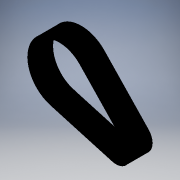
# Autodesk Inventor part: ベルト
Saved by Autodesk Inventor 2022 (Build 260153000, 153)
## iProperties
Created: 2021-07-07
Part Number: ベルト
Material: 一般
Document SubType Name: Modeling
Designer: nrz71
Density: 1 g/cm^3
Appearance: 既定
Author: nrz71
Autodesk Inventor part; units mm, degrees
ref_plane "YZ Plane" through (0, 0, 0) normal (1, 0, 0) x (0, 1, 0)
ref_plane "XZ Plane" through (0, 0, 0) normal (0, 1, 0) x (-1, 0, 0)
ref_plane "XY Plane" through (0, 0, 0) normal (0, 0, 1) x (1, 0, 0)
sketch "スケッチ1" plane through (0, 0, 0) normal (0, 0, 1) x (1, 0, 0)
  circle A0 centre (0, 0) radius 4.5
  circle A1 centre (0, 0) radius 3.5
  circle A2 centre (-17.9655, 10.8739) radius 0.9295 projected
  arc A3 (-15.3759, 19.6478) -> (-15.5156, 19.8402) centre (-15.5657, 19.657) ccw projected
  arc A4 (-15.5156, 19.8402) -> (-15.828, 19.9198) centre (-17.9655, 10.8739) ccw projected
  arc A5 (-15.828, 19.9198) -> (-16.0427, 19.8177) centre (-15.8717, 19.7349) ccw projected
  arc A6 (-16.4782, 19.3076) -> (-16.0427, 19.8177) centre (-17.2354, 20.3949) ccw projected
  arc A7 (-16.5519, 19.291) -> (-16.4782, 19.3076) centre (-16.5354, 19.3896) ccw projected
  arc A8 (-16.5519, 19.291) -> (-16.9189, 19.3445) centre (-17.9655, 10.8739) ccw projected
  arc A9 (-16.9848, 19.3814) -> (-16.9189, 19.3445) centre (-16.9067, 19.4437) ccw projected
  arc A10 (-17.2567, 19.9945) -> (-16.9848, 19.3814) centre (-15.9489, 20.2075) ccw projected
  arc A11 (-17.2567, 19.9945) -> (-17.4334, 20.1537) centre (-17.4442, 19.964) ccw projected
  arc A12 (-17.4334, 20.1537) -> (-17.7555, 20.1665) centre (-17.9655, 10.8739) ccw projected
  arc A13 (-17.7555, 20.1665) -> (-17.9443, 20.022) centre (-17.7598, 19.9766) ccw projected
  arc A14 (-18.2642, 19.4325) -> (-17.9443, 20.022) centre (-19.2309, 20.3387) ccw projected
  arc A15 (-18.3328, 19.401) -> (-18.2642, 19.4325) centre (-18.3371, 19.5009) ccw projected
  arc A16 (-18.3328, 19.401) -> (-18.7029, 19.377) centre (-17.9655, 10.8739) ccw projected
  arc A17 (-18.7751, 19.3994) -> (-18.7029, 19.377) centre (-18.7116, 19.4766) ccw projected
  arc A18 (-19.1685, 19.9426) -> (-18.7751, 19.3994) centre (-17.9336, 20.4228) ccw projected
  arc A19 (-19.1685, 19.9426) -> (-19.3744, 20.0615) centre (-19.3456, 19.8737) ccw projected
  arc A20 (-19.3744, 20.0615) -> (-19.6921, 20.0071) centre (-17.9655, 10.8739) ccw projected
  arc A21 (-19.6921, 20.0071) -> (-19.8467, 19.8265) centre (-19.6568, 19.8204) ccw projected
  arc A22 (-20.0371, 19.1834) -> (-19.8467, 19.8265) centre (-21.171, 19.8688) ccw projected
  arc A23 (-20.0977, 19.1383) -> (-20.0371, 19.1834) centre (-20.1227, 19.2351) ccw projected
  arc A24 (-20.0977, 19.1383) -> (-20.4547, 19.0378) centre (-17.9655, 10.8739) ccw projected
  arc A25 (-20.5299, 19.0447) -> (-20.4547, 19.0378) centre (-20.4839, 19.1335) ccw projected
  arc A26 (-21.0277, 19.4943) -> (-20.5299, 19.0447) centre (-19.9196, 20.2208) ccw projected
  arc A27 (-21.0277, 19.4943) -> (-21.2538, 19.5678) centre (-21.1866, 19.3901) ccw projected
  arc A28 (-21.2538, 19.5678) -> (-21.5533, 19.4485) centre (-17.9655, 10.8739) ccw projected
  arc A29 (-21.5533, 19.4485) -> (-21.667, 19.2397) centre (-21.4799, 19.2733) ccw projected
  arc A30 (-21.7195, 18.5711) -> (-21.667, 19.2397) centre (-22.9711, 19.0057) ccw projected
  arc A31 (-21.7694, 18.5144) -> (-21.7195, 18.5711) centre (-21.8139, 18.6039) ccw projected
  arc A32 (-21.7694, 18.5144) -> (-22.0977, 18.3419) centre (-17.9655, 10.8739) ccw projected
  arc A33 (-22.1727, 18.333) -> (-22.0977, 18.3419) centre (-22.1461, 18.4294) ccw projected
  arc A34 (-22.753, 18.6692) -> (-22.1727, 18.333) centre (-21.8202, 19.6103) ccw projected
  arc A35 (-22.753, 18.6692) -> (-22.9895, 18.6941) centre (-22.8868, 18.5343) ccw projected
  arc A36 (-22.9895, 18.6941) -> (-23.2577, 18.5152) centre (-17.9655, 10.8739) ccw projected
  arc A37 (-23.2577, 18.5152) -> (-23.3254, 18.2873) centre (-23.1495, 18.359) ccw projected
  arc A38 (-23.2378, 17.6224) -> (-23.3254, 18.2873) centre (-24.5525, 17.7873) ccw projected
  arc A39 (-23.2748, 17.5565) -> (-23.2378, 17.6224) centre (-23.337, 17.6348) ccw projected
  arc A40 (-23.2748, 17.5565) -> (-23.5601, 17.3196) centre (-17.9655, 10.8739) ccw projected
  arc A41 (-23.6316, 17.2953) -> (-23.5601, 17.3196) centre (-23.6256, 17.3951) ccw projected
  arc A42 (-24.2692, 17.5035) -> (-23.6316, 17.2953) centre (-23.5524, 18.6179) ccw projected
  arc A43 (-24.2692, 17.5035) -> (-24.5056, 17.4787) centre (-24.3719, 17.3437) ccw projected
  arc A44 (-24.5056, 17.4787) -> (-24.7307, 17.2479) centre (-17.9655, 10.8739) ccw projected
  arc A45 (-24.7307, 17.2479) -> (-24.7496, 17.0109) centre (-24.5924, 17.1176) ccw projected
  arc A46 (-24.5256, 16.3787) -> (-24.7496, 17.0109) centre (-25.8459, 16.2667) ccw projected
  arc A47 (-24.5482, 16.3066) -> (-24.5256, 16.3787) centre (-24.6253, 16.3703) ccw projected
  arc A48 (-24.5482, 16.3066) -> (-24.7779, 16.0155) centre (-17.9655, 10.8739) ccw projected
  arc A49 (-24.8429, 15.9769) -> (-24.7779, 16.0155) centre (-24.8578, 16.0758) ccw projected
  arc A50 (-25.5098, 16.048) -> (-24.8429, 15.9769) centre (-25.0404, 17.2871) ccw projected
  arc A51 (-25.5098, 16.048) -> (-25.7359, 15.9746) centre (-25.5771, 15.8703) ccw projected
  arc A52 (-25.7359, 15.9746) -> (-25.9081, 15.7021) centre (-17.9655, 10.8739) ccw projected
  arc A53 (-25.9081, 15.7021) -> (-25.8773, 15.4663) centre (-25.7458, 15.6034) ccw projected
  arc A54 (-25.5268, 14.8945) -> (-25.8773, 15.4663) centre (-26.7949, 14.5104) ccw projected
  arc A55 (-25.5338, 14.8193) -> (-25.5268, 14.8945) centre (-25.6225, 14.8655) ccw projected
  arc A56 (-25.5338, 14.8193) -> (-25.6981, 14.4868) centre (-17.9655, 10.8739) ccw projected
  arc A57 (-25.7535, 14.4355) -> (-25.6981, 14.4868) centre (-25.7887, 14.5291) ccw projected
  arc A58 (-26.4207, 14.3664) -> (-25.7535, 14.4355) centre (-26.2192, 15.676) ccw projected
  arc A59 (-26.4207, 14.3664) -> (-26.6266, 14.2476) centre (-26.4496, 14.1786) ccw projected
  arc A60 (-26.6266, 14.2476) -> (-26.7384, 13.9452) centre (-17.9655, 10.8739) ccw projected
  arc A61 (-26.7384, 13.9452) -> (-26.6593, 13.721) centre (-26.5591, 13.8824) ccw projected
  arc A62 (-26.1975, 13.2346) -> (-26.6593, 13.721) centre (-27.358, 12.5952) ccw projected
  arc A63 (-26.1887, 13.1595) -> (-26.1975, 13.2346) centre (-26.2851, 13.1863) ccw projected
  arc A64 (-26.1887, 13.1595) -> (-26.2803, 12.8001) centre (-17.9655, 10.8739) ccw projected
  arc A65 (-26.3239, 12.7384) -> (-26.2803, 12.8001) centre (-26.3777, 12.8227) ccw projected
  arc A66 (-26.962, 12.5321) -> (-26.3239, 12.7384) centre (-27.0372, 13.855) ccw projected
  arc A67 (-26.962, 12.5321) -> (-27.1388, 12.3731) centre (-26.9513, 12.3425) ccw projected
  arc A68 (-27.1388, 12.3731) -> (-27.1852, 12.0541) centre (-17.9655, 10.8739) ccw projected
  arc A69 (-27.1852, 12.0541) -> (-27.0612, 11.8512) centre (-26.9968, 12.03) ccw projected
  arc A70 (-26.5084, 11.4714) -> (-27.0612, 11.8512) centre (-27.5107, 10.6048) ccw projected
  arc A71 (-26.4843, 11.3999) -> (-26.5084, 11.4714) centre (-26.5841, 11.406) ccw projected
  arc A72 (-26.4843, 11.3999) -> (-26.4991, 11.0293) centre (-17.9655, 10.8739) ccw projected
  arc A73 (-26.5289, 10.9599) -> (-26.4991, 11.0293) centre (-26.599, 11.0311) ccw projected
  arc A74 (-27.1102, 10.6254) -> (-26.5289, 10.9599) centre (-27.4588, 11.9038) ccw projected
  arc A75 (-27.1102, 10.6254) -> (-27.25, 10.4331) centre (-27.0602, 10.4421) ccw projected
  arc A76 (-27.25, 10.4331) -> (-27.2291, 10.1114) centre (-17.9655, 10.8739) ccw projected
  arc A77 (-27.2291, 10.1114) -> (-27.0657, 9.9388) centre (-27.0398, 10.127) ccw projected
  arc A78 (-26.446, 9.6822) -> (-27.0657, 9.9388) centre (-27.2461, 8.6261) ccw projected
  arc A79 (-26.4075, 9.6172) -> (-26.446, 9.6822) centre (-26.5064, 9.6025) ccw projected
  arc A80 (-26.4075, 9.6172) -> (-26.3449, 9.2517) centre (-17.9655, 10.8739) ccw projected
  arc A81 (-26.3596, 9.1776) -> (-26.3449, 9.2517) centre (-26.4431, 9.2327) ccw projected
  arc A82 (-26.8587, 8.7296) -> (-26.3596, 9.1776) centre (-27.4654, 9.9075) ccw projected
  arc A83 (-26.8587, 8.7296) -> (-26.9555, 8.5124) centre (-26.7717, 8.5606) ccw projected
  arc A84 (-26.9555, 8.5124) -> (-26.8682, 8.202) centre (-17.9655, 10.8739) ccw projected
  arc A85 (-26.8682, 8.202) -> (-26.6724, 8.0672) centre (-26.6862, 8.2567) ccw projected
  arc A86 (-26.0129, 7.9451) -> (-26.6724, 8.0672) centre (-26.576, 6.7457) ccw projected
  arc A87 (-25.9617, 7.8895) -> (-26.0129, 7.9451) centre (-26.0554, 7.8545) ccw projected
  arc A88 (-25.9617, 7.8895) -> (-25.8245, 7.5449) centre (-17.9655, 10.8739) ccw projected
  arc A89 (-25.8235, 7.4694) -> (-25.8245, 7.5449) centre (-25.9166, 7.5059) ccw projected
  arc A90 (-26.2185, 6.9274) -> (-25.8235, 7.4694) centre (-27.0569, 7.9534) ccw projected
  arc A91 (-26.2185, 6.9274) -> (-26.268, 6.6948) centre (-26.0983, 6.7803) ccw projected
  arc A92 (-26.268, 6.6948) -> (-26.1181, 6.4094) centre (-17.9655, 10.8739) ccw projected
  arc A93 (-26.1181, 6.4094) -> (-25.8986, 6.3182) centre (-25.9515, 6.5007) ccw projected
  arc A94 (-25.2281, 6.3359) -> (-25.8986, 6.3182) centre (-25.5295, 5.0457) ccw projected
  arc A95 (-25.1665, 6.2922) -> (-25.2281, 6.3359) centre (-25.2508, 6.2385) ccw projected
  arc A96 (-25.1665, 6.2922) -> (-24.9606, 5.9837) centre (-17.9655, 10.8739) ccw projected
  arc A97 (-24.9439, 5.91) -> (-24.9606, 5.9837) centre (-25.0426, 5.9264) ccw projected
  arc A98 (-25.2177, 5.2977) -> (-24.9439, 5.91) centre (-26.2511, 6.127) ccw projected
  arc A99 (-25.2177, 5.2977) -> (-25.2177, 5.06) centre (-25.0695, 5.1788) ccw projected
  arc A100 (-25.2177, 5.06) -> (-25.0118, 4.812) centre (-17.9655, 10.8739) ccw projected
  arc A101 (-25.0118, 4.812) -> (-24.778, 4.7684) centre (-24.8677, 4.9359) ccw projected
  arc A102 (-24.1259, 4.9251) -> (-24.778, 4.7684) centre (-24.1525, 3.6004) ccw projected
  arc A103 (-24.0565, 4.8952) -> (-24.1259, 4.9251) centre (-24.1279, 4.8251) ccw projected
  arc A104 (-24.0565, 4.8952) -> (-23.791, 4.6362) centre (-17.9655, 10.8739) ccw projected
  arc A105 (-23.7594, 4.5676) -> (-23.791, 4.6362) centre (-23.8593, 4.5631) ccw projected
  arc A106 (-23.8998, 3.9118) -> (-23.7594, 4.5676) centre (-25.0831, 4.5081) ccw projected
  arc A107 (-23.8998, 3.9118) -> (-23.8505, 3.6792) centre (-23.7302, 3.8263) ccw projected
  arc A108 (-23.8505, 3.6792) -> (-23.5974, 3.4794) centre (-17.9655, 10.8739) ccw projected
  arc A109 (-23.5974, 3.4794) -> (-23.3597, 3.4854) centre (-23.4823, 3.6306) ccw projected
  arc A110 (-22.7544, 3.7743) -> (-23.3597, 3.4854) centre (-22.505, 2.473) ccw projected
  arc A111 (-22.6804, 3.7594) -> (-22.7544, 3.7743) centre (-22.7356, 3.6761) ccw projected
  arc A112 (-22.6804, 3.7594) -> (-22.3669, 3.5613) centre (-17.9655, 10.8739) ccw projected
  arc A113 (-22.3216, 3.5008) -> (-22.3669, 3.5613) centre (-22.4184, 3.4756) ccw projected
  arc A114 (-22.3227, 2.8301) -> (-22.3216, 3.5008) centre (-23.604, 3.1674) ccw projected
  arc A115 (-22.3227, 2.8301) -> (-22.226, 2.6129) centre (-22.1389, 2.7817) ccw projected
  arc A116 (-22.226, 2.6129) -> (-21.937, 2.4701) centre (-17.9655, 10.8739) ccw projected
  arc A117 (-21.937, 2.4701) -> (-21.7057, 2.5253) centre (-21.8558, 2.6419) ccw projected
  arc A118 (-21.1737, 2.9337) -> (-21.7057, 2.5253) centre (-20.6592, 1.7127) ccw projected
  arc A119 (-21.0982, 2.9346) -> (-21.1737, 2.9337) centre (-21.1349, 2.8416) ccw projected
  arc A120 (-21.0982, 2.9346) -> (-20.7503, 2.806) centre (-17.9655, 10.8739) ccw projected
  arc A121 (-20.6935, 2.7562) -> (-20.7503, 2.806) centre (-20.7829, 2.7115) ccw projected
  arc A122 (-20.555, 2.1) -> (-20.6935, 2.7562) centre (-21.8785, 2.1635) ccw projected
  arc A123 (-20.555, 2.1) -> (-20.4153, 1.9076) centre (-20.3653, 2.0908) ccw projected
  arc A124 (-20.4153, 1.9076) -> (-20.1029, 1.828) centre (-17.9655, 10.8739) ccw projected
  arc A125 (-20.1029, 1.828) -> (-19.8882, 1.9301) centre (-20.0592, 2.0129) ccw projected
  arc A126 (-19.4527, 2.4402) -> (-19.8882, 1.9301) centre (-18.6956, 1.3529) ccw projected
  arc A127 (-19.379, 2.4568) -> (-19.4527, 2.4402) centre (-19.3956, 2.3581) ccw projected
  arc A128 (-19.379, 2.4568) -> (-19.012, 2.4033) centre (-17.9655, 10.8739) ccw projected
  arc A129 (-18.9461, 2.3664) -> (-19.012, 2.4033) centre (-19.0243, 2.3041) ccw projected
  arc A130 (-18.6742, 1.7533) -> (-18.9461, 2.3664) centre (-19.982, 1.5402) ccw projected
  arc A131 (-18.6742, 1.7533) -> (-18.4976, 1.5941) centre (-18.4867, 1.7838) ccw projected
  arc A132 (-18.4976, 1.5941) -> (-18.1755, 1.5813) centre (-17.9655, 10.8739) ccw projected
  arc A133 (-18.1755, 1.5813) -> (-17.9867, 1.7258) centre (-18.1712, 1.7712) ccw projected
  arc A134 (-17.6668, 2.3153) -> (-17.9867, 1.7258) centre (-16.7001, 1.4091) ccw projected
  arc A135 (-17.5981, 2.3468) -> (-17.6668, 2.3153) centre (-17.5938, 2.2469) ccw projected
  arc A136 (-17.5981, 2.3468) -> (-17.228, 2.3708) centre (-17.9655, 10.8739) ccw projected
  arc A137 (-17.1559, 2.3484) -> (-17.228, 2.3708) centre (-17.2194, 2.2712) ccw projected
  arc A138 (-16.7625, 1.8052) -> (-17.1559, 2.3484) centre (-17.9974, 1.325) ccw projected
  arc A139 (-16.7625, 1.8052) -> (-16.5566, 1.6863) centre (-16.5854, 1.8741) ccw projected
  arc A140 (-16.5566, 1.6863) -> (-16.2388, 1.7407) centre (-17.9655, 10.8739) ccw projected
  arc A141 (-16.2388, 1.7407) -> (-16.0842, 1.9213) centre (-16.2741, 1.9274) ccw projected
  arc A142 (-15.8939, 2.5644) -> (-16.0842, 1.9213) centre (-14.7599, 1.879) ccw projected
  arc A143 (-15.8333, 2.6095) -> (-15.8939, 2.5644) centre (-15.8083, 2.5127) ccw projected
  arc A144 (-15.8333, 2.6095) -> (-15.4762, 2.71) centre (-17.9655, 10.8739) ccw projected
  arc A145 (-15.401, 2.7031) -> (-15.4762, 2.71) centre (-15.4471, 2.6143) ccw projected
  arc A146 (-14.9033, 2.2535) -> (-15.401, 2.7031) centre (-16.0113, 1.527) ccw projected
  arc A147 (-14.9033, 2.2535) -> (-14.6772, 2.18) centre (-14.7444, 2.3577) ccw projected
  arc A148 (-14.6772, 2.18) -> (-14.3777, 2.2992) centre (-17.9655, 10.8739) ccw projected
  arc A149 (-14.3777, 2.2992) -> (-14.264, 2.5081) centre (-14.451, 2.4745) ccw projected
  arc A150 (-14.2115, 3.1767) -> (-14.264, 2.5081) centre (-12.9598, 2.7421) ccw projected
  arc A151 (-14.1616, 3.2334) -> (-14.2115, 3.1767) centre (-14.117, 3.1439) ccw projected
  arc A152 (-14.1616, 3.2334) -> (-13.8333, 3.4059) centre (-17.9655, 10.8739) ccw projected
  arc A153 (-13.7583, 3.4148) -> (-13.8333, 3.4059) centre (-13.7849, 3.3184) ccw projected
  arc A154 (-13.1779, 3.0786) -> (-13.7583, 3.4148) centre (-14.1107, 2.1375) ccw projected
  arc A155 (-13.1779, 3.0786) -> (-12.9415, 3.0536) centre (-13.0442, 3.2135) ccw projected
  arc A156 (-12.9415, 3.0536) -> (-12.6733, 3.2326) centre (-17.9655, 10.8739) ccw projected
  arc A157 (-12.6733, 3.2326) -> (-12.6055, 3.4605) centre (-12.7815, 3.3888) ccw projected
  arc A158 (-12.6932, 4.1254) -> (-12.6055, 3.4605) centre (-11.3785, 3.9605) ccw projected
  arc A159 (-12.6562, 4.1913) -> (-12.6932, 4.1254) centre (-12.594, 4.113) ccw projected
  arc A160 (-12.6562, 4.1913) -> (-12.3709, 4.4282) centre (-17.9655, 10.8739) ccw projected
  arc A161 (-12.2994, 4.4525) -> (-12.3709, 4.4282) centre (-12.3053, 4.3527) ccw projected
  arc A162 (-11.6618, 4.2443) -> (-12.2994, 4.4525) centre (-12.3785, 3.1299) ccw projected
  arc A163 (-11.6618, 4.2443) -> (-11.4253, 4.2691) centre (-11.559, 4.4041) ccw projected
  arc A164 (-11.4253, 4.2691) -> (-11.2002, 4.4999) centre (-17.9655, 10.8739) ccw projected
  arc A165 (-11.2002, 4.4999) -> (-11.1813, 4.7369) centre (-11.3385, 4.6302) ccw projected
  arc A166 (-11.4053, 5.3691) -> (-11.1813, 4.7369) centre (-10.0851, 5.4811) ccw projected
  arc A167 (-11.3828, 5.4412) -> (-11.4053, 5.3691) centre (-11.3057, 5.3775) ccw projected
  arc A168 (-11.3828, 5.4412) -> (-11.153, 5.7323) centre (-17.9655, 10.8739) ccw projected
  arc A169 (-11.0881, 5.7709) -> (-11.153, 5.7323) centre (-11.0732, 5.672) ccw projected
  arc A170 (-10.4212, 5.6998) -> (-11.0881, 5.7709) centre (-10.8906, 4.4607) ccw projected
  arc A171 (-10.4212, 5.6998) -> (-10.195, 5.7732) centre (-10.3539, 5.8775) ccw projected
  arc A172 (-10.195, 5.7732) -> (-10.0228, 6.0457) centre (-17.9655, 10.8739) ccw projected
  arc A173 (-10.0228, 6.0457) -> (-10.0536, 6.2815) centre (-10.1852, 6.1444) ccw projected
  arc A174 (-10.4042, 6.8533) -> (-10.0536, 6.2815) centre (-9.136, 7.2374) ccw projected
  arc A175 (-10.3971, 6.9285) -> (-10.4042, 6.8533) centre (-10.3084, 6.8823) ccw projected
  arc A176 (-10.3971, 6.9285) -> (-10.2329, 7.261) centre (-17.9655, 10.8739) ccw projected
  arc A177 (-10.1774, 7.3123) -> (-10.2329, 7.261) centre (-10.1423, 7.2187) ccw projected
  arc A178 (-9.5103, 7.3814) -> (-10.1774, 7.3123) centre (-9.7118, 6.0718) ccw projected
  arc A179 (-9.5103, 7.3814) -> (-9.3043, 7.5002) centre (-9.4814, 7.5692) ccw projected
  arc A180 (-9.3043, 7.5002) -> (-9.1926, 7.8026) centre (-17.9655, 10.8739) ccw projected
  arc A181 (-9.1926, 7.8026) -> (-9.2717, 8.0268) centre (-9.3719, 7.8654) ccw projected
  arc A182 (-9.7335, 8.5132) -> (-9.2717, 8.0268) centre (-8.5729, 9.1526) ccw projected
  arc A183 (-9.7422, 8.5883) -> (-9.7335, 8.5132) centre (-9.6459, 8.5615) ccw projected
  arc A184 (-9.7422, 8.5883) -> (-9.6507, 8.9477) centre (-17.9655, 10.8739) ccw projected
  arc A185 (-9.6071, 9.0094) -> (-9.6507, 8.9477) centre (-9.5533, 8.9251) ccw projected
  arc A186 (-8.9689, 9.2156) -> (-9.6071, 9.0094) centre (-8.8937, 7.8928) ccw projected
  arc A187 (-8.9689, 9.2156) -> (-8.7922, 9.3747) centre (-8.9797, 9.4053) ccw projected
  arc A188 (-8.7922, 9.3747) -> (-8.7457, 9.6937) centre (-17.9655, 10.8739) ccw projected
  arc A189 (-8.7457, 9.6937) -> (-8.8697, 9.8966) centre (-8.9342, 9.7178) ccw projected
  arc A190 (-9.4225, 10.2764) -> (-8.8697, 9.8966) centre (-8.4203, 11.143) ccw projected
  arc A191 (-9.4467, 10.3479) -> (-9.4225, 10.2764) centre (-9.3469, 10.3418) ccw projected
  arc A192 (-9.4467, 10.3479) -> (-9.4319, 10.7185) centre (-17.9655, 10.8739) ccw projected
  arc A193 (-9.4021, 10.7879) -> (-9.4319, 10.7185) centre (-9.3319, 10.7167) ccw projected
  arc A194 (-8.8207, 11.1224) -> (-9.4021, 10.7879) centre (-8.4722, 9.844) ccw projected
  arc A195 (-8.8207, 11.1224) -> (-8.6809, 11.3147) centre (-8.8707, 11.3057) ccw projected
  arc A196 (-8.6809, 11.3147) -> (-8.7018, 11.6364) centre (-17.9655, 10.8739) ccw projected
  arc A197 (-8.7018, 11.6364) -> (-8.8653, 11.809) centre (-8.8912, 11.6208) ccw projected
  arc A198 (-9.485, 12.0656) -> (-8.8653, 11.809) centre (-8.6848, 13.1217) ccw projected
  arc A199 (-9.5235, 12.1306) -> (-9.485, 12.0656) centre (-9.4246, 12.1453) ccw projected
  arc A200 (-9.5235, 12.1306) -> (-9.5861, 12.4961) centre (-17.9655, 10.8739) ccw projected
  arc A201 (-9.5713, 12.5702) -> (-9.5861, 12.4961) centre (-9.4879, 12.5151) ccw projected
  arc A202 (-9.0722, 13.0182) -> (-9.5713, 12.5702) centre (-8.4655, 11.8403) ccw projected
  arc A203 (-9.0722, 13.0182) -> (-8.9755, 13.2354) centre (-9.1592, 13.1872) ccw projected
  arc A204 (-8.9755, 13.2354) -> (-9.0628, 13.5458) centre (-17.9655, 10.8739) ccw projected
  arc A205 (-9.0628, 13.5458) -> (-9.2586, 13.6806) centre (-9.2448, 13.4911) ccw projected
  arc A206 (-9.9181, 13.8027) -> (-9.2586, 13.6806) centre (-9.355, 15.0021) ccw projected
  arc A207 (-9.9693, 13.8583) -> (-9.9181, 13.8027) centre (-9.8756, 13.8933) ccw projected
  arc A208 (-9.9693, 13.8583) -> (-10.1065, 14.2029) centre (-17.9655, 10.8739) ccw projected
  arc A209 (-10.1075, 14.2784) -> (-10.1065, 14.2029) centre (-10.0144, 14.2419) ccw projected
  arc A210 (-9.7124, 14.8204) -> (-10.1075, 14.2784) centre (-8.874, 13.7944) ccw projected
  arc A211 (-9.7124, 14.8204) -> (-9.6629, 15.0529) centre (-9.8326, 14.9675) ccw projected
  arc A212 (-9.6629, 15.0529) -> (-9.8128, 15.3383) centre (-17.9655, 10.8739) ccw projected
  arc A213 (-9.8128, 15.3383) -> (-10.0324, 15.4296) centre (-9.9795, 15.2471) ccw projected
  arc A214 (-10.7029, 15.4119) -> (-10.0324, 15.4296) centre (-10.4014, 16.7021) ccw projected
  arc A215 (-10.7645, 15.4556) -> (-10.7029, 15.4119) centre (-10.6801, 15.5093) ccw projected
  arc A216 (-10.7645, 15.4556) -> (-10.9703, 15.7641) centre (-17.9655, 10.8739) ccw projected
  arc A217 (-10.987, 15.8378) -> (-10.9703, 15.7641) centre (-10.8884, 15.8214) ccw projected
  arc A218 (-10.7133, 16.4501) -> (-10.987, 15.8378) centre (-9.6799, 15.6208) ccw projected
  arc A219 (-10.7133, 16.4501) -> (-10.7132, 16.6878) centre (-10.8615, 16.569) ccw projected
  arc A220 (-10.7132, 16.6878) -> (-10.9192, 16.9358) centre (-17.9655, 10.8739) ccw projected
  arc A221 (-10.9192, 16.9358) -> (-11.1529, 16.9794) centre (-11.0632, 16.8119) ccw projected
  arc A222 (-11.8051, 16.8227) -> (-11.1529, 16.9794) centre (-11.7785, 18.1474) ccw projected
  arc A223 (-11.8744, 16.8526) -> (-11.8051, 16.8227) centre (-11.8031, 16.9227) ccw projected
  arc A224 (-11.8744, 16.8526) -> (-12.1399, 17.1116) centre (-17.9655, 10.8739) ccw projected
  arc A225 (-12.1716, 17.1802) -> (-12.1399, 17.1116) centre (-12.0717, 17.1847) ccw projected
  arc A226 (-12.0311, 17.836) -> (-12.1716, 17.1802) centre (-10.8479, 17.2397) ccw projected
  arc A227 (-12.0311, 17.836) -> (-12.0805, 18.0686) centre (-12.2008, 17.9215) ccw projected
  arc A228 (-12.0805, 18.0686) -> (-12.3335, 18.2684) centre (-17.9655, 10.8739) ccw projected
  arc A229 (-12.3335, 18.2684) -> (-12.5712, 18.2624) centre (-12.4486, 18.1172) ccw projected
  arc A230 (-13.1765, 17.9735) -> (-12.5712, 18.2624) centre (-13.4259, 19.2748) ccw projected
  arc A231 (-13.2506, 17.9884) -> (-13.1765, 17.9735) centre (-13.1953, 18.0717) ccw projected
  arc A232 (-13.2506, 17.9884) -> (-13.5641, 18.1865) centre (-17.9655, 10.8739) ccw projected
  arc A233 (-13.6093, 18.247) -> (-13.5641, 18.1865) centre (-13.5125, 18.2722) ccw projected
  arc A234 (-13.6083, 18.9177) -> (-13.6093, 18.247) centre (-12.3269, 18.5804) ccw projected
  arc A235 (-13.6083, 18.9177) -> (-13.7049, 19.1349) centre (-13.792, 18.9661) ccw projected
  arc A236 (-13.7049, 19.1349) -> (-13.994, 19.2777) centre (-17.9655, 10.8739) ccw projected
  arc A237 (-13.994, 19.2777) -> (-14.2252, 19.2225) centre (-14.0752, 19.1059) ccw projected
  arc A238 (-14.7573, 18.8141) -> (-14.2252, 19.2225) centre (-15.2718, 20.0351) ccw projected
  arc A239 (-14.8328, 18.8132) -> (-14.7573, 18.8141) centre (-14.7961, 18.9062) ccw projected
  arc A240 (-14.8328, 18.8132) -> (-15.1807, 18.9418) centre (-17.9655, 10.8739) ccw projected
  arc A241 (-15.2375, 18.9916) -> (-15.1807, 18.9418) centre (-15.148, 19.0363) ccw projected
  arc A242 (-15.3759, 19.6478) -> (-15.2375, 18.9916) centre (-14.0524, 19.5843) ccw projected
  circle A243 centre (-17.9655, 10.8739) radius 9
  circle A244 centre (-17.9655, 10.8739) radius 10
  line L0 (3.2571, 3.1051) -> (-10.7276, 17.7741)
  line L1 (-1.2405, -4.3256) -> (-20.7222, 1.2614)
  line L2 (2.5333, 2.4151) -> (-11.4514, 17.0841)
  line L3 (-0.9648, -3.3644) -> (-20.4465, 2.2226)
  point P0 (-0.9474, -3.3693)
  point P1 (-20.5567, 2.255)
  point P2 (-21.6036, 2.642)
  point P3 (-22.292, 2.9821)
  point P4 (-23.2356, 3.5783)
  point P5 (-23.8383, 4.0541)
  point P6 (-24.6373, 4.8335)
  point P7 (-25.1279, 5.4241)
  point P8 (-25.7474, 6.3526)
  point P9 (-26.1044, 7.0324)
  point P10 (-26.5174, 8.0694)
  point P11 (-26.7253, 8.8085)
  point P12 (-26.9136, 9.9087)
  point P13 (-26.9633, 10.6749)
  point P14 (-26.9187, 11.7902)
  point P15 (-26.808, 12.55)
  point P16 (-26.5326, 13.6317)
  point P17 (-26.2663, 14.3518)
  point P18 (-25.772, 15.3526)
  point P19 (-25.3618, 16.0017)
  point P20 (-24.6702, 16.8778)
  point P21 (-24.1341, 17.4274)
  point P22 (-23.2754, 18.1406)
  point P23 (-22.6367, 18.5667)
  point P24 (-21.6486, 19.0858)
  point P25 (-20.9352, 19.3698)
  point P26 (-19.8607, 19.6721)
  point P27 (-19.1039, 19.8016)
  point P28 (-17.9901, 19.8739)
  point P29 (-17.2229, 19.8432)
  point P30 (-16.1183, 19.6823)
  point P31 (-15.3743, 19.4928)
  point P32 (-14.3273, 19.1058)
  point P33 (-13.6389, 18.7657)
  point P34 (-12.6953, 18.1695)
  point P35 (-12.0927, 17.6937)
  point P36 (-11.2907, 16.9155)
  point P37 (-10.7718, 16.3713)
  point P38 (-19.8126, 2.0655)
  point P39 (-10.1836, 15.3952)
  point P40 (-9.8265, 14.7154)
  point P41 (-9.4136, 13.6784)
  point P42 (-9.2057, 12.9393)
  point P43 (-9.0174, 11.8391)
  point P44 (-8.9677, 11.0729)
  point P45 (-9.0122, 9.9576)
  point P46 (-9.1229, 9.1978)
  point P47 (-9.3984, 8.1161)
  point P48 (-9.6646, 7.396)
  point P49 (-10.159, 6.3952)
  point P50 (-10.5691, 5.7461)
  point P51 (-11.2607, 4.87)
  point P52 (-11.7969, 4.3204)
  point P53 (-12.6555, 3.6072)
  point P54 (-13.2942, 3.1811)
  point P55 (-14.2824, 2.662)
  point P56 (-14.9957, 2.378)
  point P57 (-16.0702, 2.0757)
  point P58 (-16.827, 1.9462)
  point P59 (-17.9409, 1.8739)
  point P60 (-18.7081, 1.9046)
  point P61 (-10.8031, 16.3237)
  point P62 (-11.2937, 16.9143)
  point P63 (-19.8257, 2.0446)
  dimension "d2" = 18
  dimension "d0" = 9
  dimension "d1" = 7
  dimension "d3" = 20
  constraints: 8 end point, 7 point on circle, 6 tangent, 4 coincident, 3 centre point, 5 other
  measures "d0" diameter of A0
  measures "d1" diameter of A1
  measures "d3" diameter of A244
extrude "押し出し1" add sketch "スケッチ1" along normal blind 7 contours A0 L3 A1 L2 | A0 L2 A244 L0 | L1 A244 L3 A0 | A244 L2 A218 A219 A220 A221 A222 A243 A226 A227 A228 A229 A230 A234 A235 A236 A237 A238 A242 A3 A4 A5 A6 A10 A11 A12 A13 A14 A18 A19 A20 A21 A22 A26 A27 A28 A29 A30 A34 A35 A36 A37 A38 A42 A43 A44 A45 A46 A50 A51 A52 A53 A54 A58 A59 A60 A61 A62 A66 A67 A68 A69 A70 A74 A75 A76 A77 A78 A82 A83 A84 A85 A86 A90 A91 A92 A93 A94 A98 A99 A100 A101 A102 A106 A107 A108 A109 A110 A114 A115 A116 A117 A118 A122 A123 A124 A125 A126 L3 A131 A132 | L2 A222 A221 A220 A219 A218 | A132 A131 L3 | L3 A243 A126 | A126 A125 A124 A123 A122 A243 L3 | A243 A230 A229 A228 A227 A226 | A243 A238 A237 A236 A235 A234 | A118 A117 A116 A115 A114 A243 | A243 A6 A5 A4 A3 A242 | A110 A109 A108 A107 A106 A243 | A243 A14 A13 A12 A11 A10 | A102 A101 A100 A99 A98 A243 | A243 A22 A21 A20 A19 A18 | A94 A93 A92 A91 A90 A243 | A243 A30 A29 A28 A27 A26 | A86 A85 A84 A83 A82 A243 | A243 A38 A37 A36 A35 A34 | A78 A77 A76 A75 A74 A243 | A243 A46 A45 A44 A43 A42 | A70 A69 A68 A67 A66 A243 | A243 A54 A53 A52 A51 A50 | A62 A61 A60 A59 A58 A243 picked at (-2.5525, -3.0984)
equation "\"d4\" = d1"
